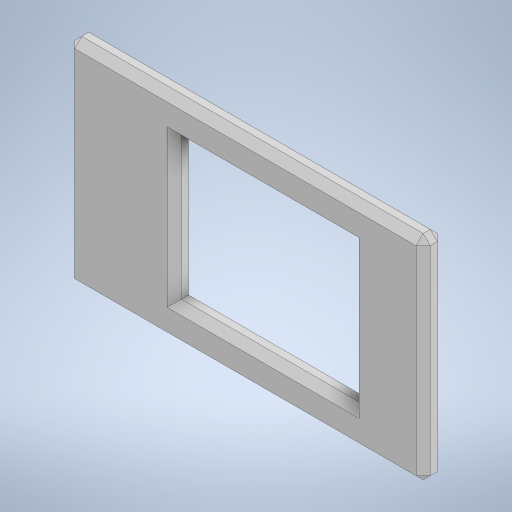
# Autodesk Inventor part: colorlabel
Saved by Autodesk Inventor 2024 (Build 280153000, 153)
## iProperties
Created: 2026-05-14
Part Number: colorlabel
Material: Generic
Document SubType Name: Modeling
Designer: janst
Density: 1 g/cm^3
Appearance: Default
Author: janst
Autodesk Inventor part; units mm, degrees
ref_plane "YZ Plane" through (0, 0, 0) normal (1, 0, 0) x (0, 1, 0)
ref_plane "XZ Plane" through (0, 0, 0) normal (0, 1, 0) x (-1, 0, 0)
ref_plane "XY Plane" through (0, 0, 0) normal (0, 0, 1) x (1, 0, 0)
sketch "Sketch1" plane through (0, 0, 0) normal (0, 0, 1) x (1, 0, 0)
  line L0 (25, -15) -> (-25, -15)
  line L1 (-25, -15) -> (-25, 15)
  line L2 (-25, 15) -> (25, 15)
  line L3 (25, 15) -> (25, -15)
  line L4 (25, -15) -> (-25, 15) construction
  line L5 (-25, -15) -> (25, 15) construction
  line L6 (15, -10) -> (-10, -10)
  line L7 (-10, -10) -> (-10, 10)
  line L8 (-10, 10) -> (15, 10)
  line L9 (15, 10) -> (15, -10)
  line L10 (15, -10) -> (-10, 10) construction
  line L11 (-10, -10) -> (15, 10) construction
  point P0 (0, 0)
  point P1 (2.5, 0)
  point P2 (0, 0)
  dimension "d0" = 25
  dimension "d1" = 20
  dimension "d2" = 30
  dimension "d3" = 5
  dimension "d4" = 10
  dimension "d5" = 15
  constraints: 24 end point, 4 midpoint, 4 parallel, 2 horizontal, 2 perpendicular, 1 coincident
  measures "d0" distance of L7.end L8.end
  measures "d1" distance of L8.end L6.start
  measures "d2" distance of L2.end L0.start
  measures "d3" distance between parallel lines of L0 L6
  measures "d4" distance between parallel lines of L3 L9
  measures "d5" distance between parallel lines of L1 L7
extrude "Extrusion1" add sketch "Sketch1" along normal blind 3
chamfer "Chamfer1" distance 1 angle 45 20 edges at (0, 15, 3) (25, 0, 3) (-25, 0, 3) (0, -15, 3) (2.5, -10, 3) (-10, 0, 3) (2.5, 10, 3) (15, 0, 3) (0, 15, 0) (25, 0, 0) (0, -15, 0) (-25, 0, 0) (-25, -15, 1.5) (-25, 15, 1.5) (25, 15, 1.5) (25, -15, 1.5) (-10, 0, 0) (2.5, 10, 0) (15, 0, 0) (2.5, -10, 0)
equation "\"d3\" = -0.5 * d1 + 0.5 * d2"
body "Solid1"
